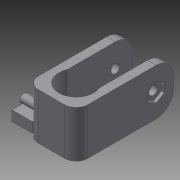
# Autodesk Inventor part: microswitch 12mm axe support
Saved by Autodesk Inventor 2015 SP1 (Build 190203100, 203)
## iProperties
Created: 2015-08-09
Part Number: microswitch 12mm axe support
Material: Generic
Document SubType Name: Modeling
Designer: ubik
Density: 1 g/cm^3
Appearance: Default
Author: ubik
Autodesk Inventor part; units mm, degrees
ref_plane "YZ Plane" through (0, 0, 0) normal (1, 0, 0) x (0, 1, 0)
ref_plane "XZ Plane" through (0, 0, 0) normal (0, 1, 0) x (-1, 0, 0)
ref_plane "XY Plane" through (0, 0, 0) normal (0, 0, 1) x (1, 0, 0)
sketch "Sketch1" plane through (0, 0, 0) normal (0, 0, 1) x (1, 0, 0)
  arc A0 (-5.5, 2.3979) -> (5.5, 2.3979) centre (0, 0) ccw
  line L0 (-8.5, 0) -> (-8.5, 25)
  line L1 (-8.5, 25) -> (-5.5, 25)
  line L2 (-5.5, 25) -> (-5.5, 2.3979)
  line L3 (5.5, 2.3979) -> (5.5, 25)
  line L4 (5.5, 25) -> (8.5, 25)
  line L5 (8.5, 25) -> (8.5, 0)
  arc A1 (-8.5, 0) -> (8.5, 0) centre (0, 0) ccw
  dimension "d0" = 12
  dimension "d2" = 25
  dimension "d4" = 3
  dimension "d5" = 3
  dimension "d6" = 8.5
  constraints: 12 end point, 4 point on circle, 2 centre point, 2 coincident, 2 point on line, 2 tangent, 1 parallel, 1 perpendicular, 1 vertical
  measures "d0" diameter of A0
  measures "d2" distance of L0.start L0.end
  measures "d4" distance between parallel lines of L2 L0
  measures "d5" distance between parallel lines of L5 L3
  measures "d6" radius of A1
extrude "Extrusion1" add sketch "Sketch1" along normal blind 16
fillet "Fillet1" radius 6 4 edges at (-7, 25, 16) (-7, 25, 0) (7, 25, 0) (7, 25, 16)
sketch "Sketch2" plane through (-8.5, 0, 0) normal (-1, 0, 0) x (0, 0, 1)
  circle A0 centre (5, -2.5) radius 1.4
  circle A1 centre (5, 7.025) radius 1.4
  line L0 (0, 0) -> (0, 19) projected
  line L1 (0, -8.5) -> (16, -8.5) projected
  dimension "d10" = 2.8
  dimension "d11" = 2.8
  dimension "d12" = 9.525
  dimension "d13" = 5
  dimension "d14" = 6
  constraints: 2 centre point
  measures "d10" diameter of A0
  measures "d11" diameter of A1
  measures "d12" distance of A1.centre A0.centre
  measures "d13" distance from line of L0 A0.centre
  measures "d14" distance from line of L1 A0.centre
extrude "Extrusion2" add sketch "Sketch2" along normal blind 7
sketch "Sketch3" plane through (0, 0, 0) normal (0, 0, -1) x (-1, 0, 0)
  line L0 (-8.5, 19) -> (-5.5, 19) projected
  line L1 (-8.5, 19) -> (-8.5, 0) projected
  arc A0 (-8.5, 0) -> (8.5, 0) centre (0, 0) ccw projected
  line L2 (8.5, 0) -> (8.5, 19) projected
  line L3 (5.5, 19) -> (8.5, 19) projected
  line L4 (5.5, 19) -> (5.5, 2.3979) projected
  arc A1 (-5.5, 2.3979) -> (5.5, 2.3979) centre (0, 0) ccw projected
  line L5 (-5.5, 2.3979) -> (-5.5, 19) projected
  line L6 (8.5, 0) -> (8.5, -8.5)
  arc A2 (-8.5, 0) -> (8.5, 0) centre (0, 0) ccw projected
  line L7 (8.5, -1.1) -> (8.5, -3.9) projected
  line L8 (8.5, -8.5) -> (-8.5, -8.5)
  line L9 (-8.5, 0) -> (-8.5, -8.5)
  line L10 (8.5, 0) -> (6, 0)
  line L11 (-8.5, 19) -> (-8.5, 0) projected
  line L12 (-6, 0) -> (-8.5, 0)
  constraints: 10 end point, 4 perpendicular, 3 tangent, 2 point on circle, 1 collinear
extrude "Extrusion3" add sketch "Sketch3" against normal up to surface (16 mm away) contours A0 L8 L9 | A0 L6 L8
fillet "Fillet2" radius 4 2 edges at (-8.5, -8.5, 8) (8.5, -8.5, 8)
hole "Hole1" at (-8.5, 19, 8) direction (1, 0, 0) diameter 3 end through all
sketch "Sketch5" plane through (8.5, 25, 10) normal (1, 0, 0) x (0, 0, -1)
  circle A0 centre (2, -6) radius 1.5 projected
  line L0 (10, -29.5) -> (-6, -29.5) projected
  line L1 (10, -6) -> (10, -29.5) projected
  arc A1 (10, -6) -> (4, 0) centre (4, -6) ccw projected
  line L2 (4, 0) -> (0, 0) projected
  arc A2 (0, 0) -> (-6, -6) centre (0, -6) ccw projected
  line L3 (-6, -6) -> (-6, -29.5) projected
  line L4 (5.2332, -6) -> (3.6166, -8.8)
  line L5 (3.6166, -8.8) -> (0.3834, -8.8)
  line L6 (0.3834, -8.8) -> (-1.2332, -6)
  line L7 (-1.2332, -6) -> (0.3834, -3.2)
  line L8 (0.3834, -3.2) -> (3.6166, -3.2)
  line L9 (3.6166, -3.2) -> (5.2332, -6)
  point P0 (10, -25)
  dimension "d29" = 5.6
  constraints: 12 end point, 1 coincident, 13 other
  measures "d29" distance between parallel lines of L5 L8
extrude "Extrusion4" cut sketch "Sketch5" against normal blind 1 contours L4 L5 L6 L7 L8 L9
sketch "Sketch6" plane through (0, 0, 0) normal (0, 0, -1) x (-1, 0, 0)
  arc A0 (-8.5, -4.5) -> (-4.5, -8.5) centre (-4.5, -4.5) ccw projected
  line L0 (-4.5, -8.5) -> (4.5, -8.5) projected
  arc A1 (4.5, -8.5) -> (8.5, -4.5) centre (4.5, -4.5) ccw projected
  line L1 (8.5, -4.5) -> (8.5, 19) projected
  line L2 (5.5, 19) -> (8.5, 19) projected
  line L3 (5.5, 19) -> (5.5, 2.3979) projected
  arc A2 (-5.5, 2.3979) -> (5.5, 2.3979) centre (0, 0) ccw projected
  line L4 (-5.5, 2.3979) -> (-5.5, 19) projected
  line L5 (-8.5, 19) -> (-5.5, 19) projected
  line L6 (-8.5, 19) -> (-8.5, -4.5) projected
  line L7 (15.5, 5.625) -> (15.5, 8.425) projected
  line L8 (8.5, 8.425) -> (8.5, 5.625) projected
  line L9 (15.5, -3.9) -> (15.5, -1.1) projected
  line L10 (8.5, -1.1) -> (8.5, -3.9) projected
  line L11 (8.5, 8.425) -> (15.5, 8.425)
  line L12 (8.5, 5.625) -> (15.5, 5.625)
  line L13 (8.5, -1.1) -> (15.5, -1.1) projected
  line L14 (8.5, -3.9) -> (15.5, -3.9) projected
  line L15 (8.5, 10) -> (15.5, 10)
  line L16 (15.5, 10) -> (15.5, 4)
  line L17 (15.5, 4) -> (8.5, 4)
  line L18 (8.5, 4) -> (8.5, 10)
  line L19 (8.5, 19) -> (8.5, -4.5) projected
  line L20 (8.5, 1) -> (15.5, 1)
  line L21 (15.5, 1) -> (15.5, -6.597)
  line L22 (15.5, -6.597) -> (8.5, -6.597)
  line L23 (8.5, -6.597) -> (8.5, 1)
  constraints: 20 end point, 4 coincident, 4 parallel, 2 horizontal, 2 perpendicular, 2 point on line, 2 other
extrude "Extrusion6" add sketch "Sketch6" against normal blind 3.5 contours L1 L14 L21 L22 L23 | L1 L20 L21 L13 | L1 L12 L16 L17 | L15 L16 L11 L1
sketch "Sketch7" plane through (0, 0, 3.5) normal (0, 0, 1) x (1, 0, 0)
  line L0 (-8.5, 5.625) -> (-15.5, 5.625)
  line L1 (-15.5, 5.625) -> (-15.5, 4)
  line L2 (-15.5, 4) -> (-8.5, 4)
  line L3 (-8.5, 5.625) -> (-8.5, 4)
  line L4 (-15.5, 8.425) -> (-8.5, 8.425)
  line L5 (-8.5, 10) -> (-8.5, 5.625)
  line L6 (-8.5, 10) -> (-15.5, 10)
  line L7 (-15.5, 10) -> (-15.5, 5.625)
  line L8 (-15.5, -1.1) -> (-8.5, -1.1)
  line L9 (-8.5, 1) -> (-8.5, -3.9)
  line L10 (-8.5, 1) -> (-15.5, 1) projected
  line L11 (-15.5, 1) -> (-15.5, -3.9)
  line L12 (-8.5, -3.9) -> (-15.5, -3.9)
  line L13 (-15.5, -3.9) -> (-15.5, -6.597)
  line L14 (-15.5, -6.597) -> (-8.5, -6.597) projected
  line L15 (-8.5, -6.597) -> (-8.5, -4.5)
  line L16 (-8.5, -3.9) -> (-8.5, -4.5) projected
  line L17 (-8.5, 8.425) -> (-7, 6)
  line L18 (-8.5, 5.625) -> (-15.5, 5.625) projected
  point P0 (0, 0)
  constraints: 30 end point, 7 point on line
extrude "Extrusion7" add sketch "Sketch7" against normal blind 0.5 contours L0 L7 L4 L5 | L8 L9 L12 L11
body "Solid1"
